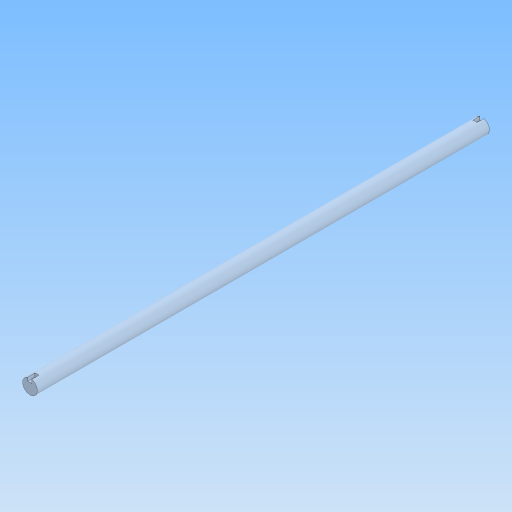
# Autodesk Inventor part: Welle
Saved by Autodesk Inventor 2024.4 (Build 284460000, 460)
## iProperties
Created: 2026-01-19
Part Number: Welle
Material: Generisch
Document SubType Name: Modeling
Designer: windows-desktop
Density: 1 g/cm^3
Appearance: Vorgabe
Mass: 374.862 g
Surface Area: 614.154 cm^2
Volume: 374.862 cm^3
Masse[kg]: 0,375 kg
Author: windows-desktop
Autodesk Inventor part; units mm, degrees
ref_plane "XZ Plane" through (0, 0, 0) normal (0, 1, 0) x (-1, 0, 0)
sketch "Skizze1" plane through (0, 0, 0) normal (0, 1, 0) x (-1, 0, 0)
  circle A0 centre (0, 0) radius 12.5
  dimension "d0" = 25
  constraints: 1 centre point, 1 coincident
  measures "d0" diameter of A0
extrude "Extrusion1" add sketch "Skizze1" along normal blind 765.83
ref_plane "Arbeitsebene1" through (-7.5, 0, 0) normal (1, 0, 0) x (0, 1, 0)
ref_plane "Arbeitsebene2" through (7.5, 0, 0) normal (1, 0, 0) x (0, 1, 0)
sketch "Skizze4" plane through (0, 765.83, 0) normal (0, 1, 0) x (1, 0, 0)
  line L0 (3.5, -16) -> (-3.5, -16)
  line L1 (-3.5, -16) -> (-3.5, -6)
  line L2 (-3.5, -6) -> (3.5, -6)
  line L3 (3.5, -6) -> (3.5, -16)
  line L4 (0, 18.2) -> (0, -21.7) construction
  line L5 (-17.5, 0) -> (17.5, 0) construction
  dimension "d15" = 6
  dimension "d16" = 10
  dimension "d17" = 7
  constraints: 8 end point, 2 parallel, 1 horizontal, 1 perpendicular, 1 other
  measures "d15" distance between parallel lines of L5 L2
  measures "d16" distance of L0.end L1.end
  measures "d17" distance of L0.start L0.end
extrude "Extrusion4" cut sketch "Skizze4" against normal blind 12
sketch "Skizze5" plane through (0, 0, 0) normal (0, -1, 0) x (1, 0, 0)
  line L0 (-3.8549, 16) -> (3.1451, 16)
  line L1 (3.1451, 16) -> (3.1451, 6)
  line L2 (3.1451, 6) -> (-3.8549, 6)
  line L3 (-3.8549, 6) -> (-3.8549, 16)
  line L4 (-17.5, 0) -> (17.5, 0) construction
  dimension "d20" = 6
  dimension "d21" = 10
  dimension "d22" = 7
  constraints: 8 end point, 2 parallel, 1 horizontal, 1 perpendicular
  measures "d20" distance between parallel lines of L4 L2
  measures "d21" distance of L0.end L1.end
  measures "d22" distance of L0.start L0.end
extrude "Extrusion5" cut sketch "Skizze5" against normal blind 12
equation "\"Wellensdurchmesser\" = 35"
equation "\"Wellenlänge\" = 724.33"
